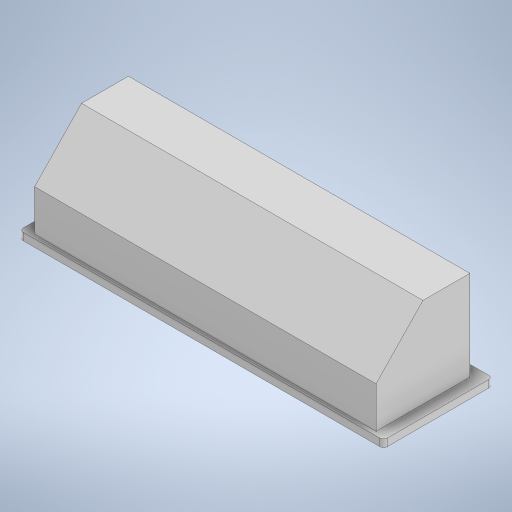
# Autodesk Inventor part: Early-944_Radio_Plug
Saved by Autodesk Inventor 2024.2 (Build 282272000, 272)
## iProperties
Created: 2024-02-12
Part Number: Early-944_Radio_Plug
Material: Generic
Document SubType Name: Modeling
Designer: Locke
Density: 1 g/cm^3
Appearance: Default
Author: Locke
Autodesk Inventor part; units mm, degrees
ref_plane "YZ Plane" through (0, 0, 0) normal (1, 0, 0) x (0, 1, 0)
ref_plane "XZ Plane" through (0, 0, 0) normal (0, 1, 0) x (-1, 0, 0)
ref_plane "XY Plane" through (0, 0, 0) normal (0, 0, 1) x (1, 0, 0)
sketch "Sketch1" plane through (0, 0, 0) normal (0, 0, 1) x (1, 0, 0)
  line L0 (0, 0) -> (182, 0)
  line L1 (182, 0) -> (182, 52)
  line L2 (182, 52) -> (0, 52)
  line L3 (0, 52) -> (0, 0)
  dimension "d0" = 182
  dimension "d1" = 52
  constraints: 8 end point, 2 parallel, 1 horizontal, 1 perpendicular
  measures "d0" distance of L2.end L1.end
  measures "d1" distance of L0.end L1.end
extrude "Extrusion1" add sketch "Sketch1" along normal blind 50
sketch "Sketch2" plane through (182, 0, 0) normal (1, 0, 0) x (0, 0, -1)
  line L0 (0, 52) -> (-50, 52) projected
  line L1 (-25, 52) -> (-50, 26)
  line L2 (-50, 0) -> (-50, 52) projected
  line L3 (-25, 52) -> (-50, 52)
  line L4 (-50, 52) -> (-50, 26)
  point P0 (0, 0)
  constraints: 6 end point, 2 midpoint, 1 collinear, 1 horizontal
extrude "Extrusion2" cut sketch "Sketch2" against normal through all
sketch "Sketch3" plane through (0, 0, 0) normal (0, -1, 0) x (1, 0, 0)
  line L0 (0, 50) -> (182, 50) projected
  line L1 (182, 0) -> (0, 0)
  line L2 (0, 0) -> (0, 50)
  line L3 (0, 50) -> (182, 50)
  line L4 (182, 50) -> (182, 0)
  line L5 (-6, -6) -> (188, -6)
  line L6 (188, -6) -> (188, 52)
  line L7 (-6, 52) -> (-6, -6)
  line L8 (182, 50) -> (0, 50)
  line L9 (188, 52) -> (-6, 52)
  dimension "d6" = 6
  constraints: 18 end point, 3 parallel, 3 perpendicular, 1 horizontal, 1 point on line
  measures "d6" distance between parallel lines of L1 L5
extrude "Extrusion3" add sketch "Sketch3" against normal blind 4 contours L0 L4 L1 L2 | L7 L9 L6 L5
fillet "Fillet1" radius 2 4 edges at (188, 2, -6) (188, 2, 52) (-6, 2, 52) (-6, 2, -6)
body "Solid1"
